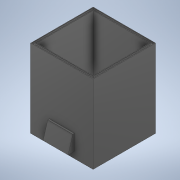
# Autodesk Inventor part: Bauteil1
Saved by Autodesk Inventor 2020 (Build 240168000, 168)
## iProperties
Created: 2021-04-07
Part Number: Bauteil1
Material: Acetalharz, Schwarz
Document SubType Name: Modeling
Designer: Julian Uhl
Density: 1.425 g/cm^3
Appearance: Glatt - Schwarz
Author: Julian Uhl
Autodesk Inventor part; units mm, degrees
ref_plane "YZ Plane" through (0, 0, 0) normal (1, 0, 0) x (0, 1, 0)
ref_plane "XZ Plane" through (0, 0, 0) normal (0, 1, 0) x (-1, 0, 0)
ref_plane "XY Plane" through (0, 0, 0) normal (0, 0, 1) x (1, 0, 0)
sketch "Skizze1" plane through (0, 0, 0) normal (0, 0, 1) x (1, 0, 0)
  line L0 (-140, 0) -> (140, 0) projected
  line L1 (0, -140) -> (0, 140) projected
  line L2 (-100, 100) -> (100, 100)
  line L3 (100, 100) -> (100, -100)
  line L4 (100, -100) -> (-100, -100)
  line L5 (-100, -100) -> (-100, 100)
  point P0 (0, 0)
  dimension "d0" = 200
  dimension "d1" = 200
  dimension "d2" = 100
  dimension "d3" = 100
  constraints: 8 end point, 2 parallel, 1 horizontal, 1 perpendicular
  measures "d0" distance between parallel lines of L3 L5
  measures "d1" distance between parallel lines of L4 L2
  measures "d2" distance between parallel lines of L0 L2
  measures "d3" distance between parallel lines of L1 L5
extrude "Extrusion1" add sketch "Skizze1" along normal blind 200
sketch "Skizze2" plane through (-100, 100, 0) normal (0, 1, 0) x (1, 0, 0)
  line L0 (10, -10) -> (190, -10)
  line L1 (190, -10) -> (190, -190)
  line L2 (190, -190) -> (10, -190)
  line L3 (10, -190) -> (10, -10)
  line L4 (0, 0) -> (0, -200) projected
  line L5 (200, 0) -> (200, -200) projected
  line L6 (200, -200) -> (0, -200) projected
  line L7 (200, 0) -> (0, 0) projected
  point P0 (100, 0)
  dimension "d6" = 10
  dimension "d7" = 10
  dimension "d8" = 10
  dimension "d9" = 10
  constraints: 8 end point, 2 parallel, 1 horizontal, 1 perpendicular
  measures "d6" distance between parallel lines of L3 L4
  measures "d7" distance between parallel lines of L5 L1
  measures "d8" distance between parallel lines of L6 L2
  measures "d9" distance between parallel lines of L0 L7
extrude "Extrusion2" cut sketch "Skizze2" against normal blind 190 contours L0 L1 L2 L3
sketch "Skizze3" plane through (-100, 100, 0) normal (0, 1, 0) x (1, 0, 0)
  line L0 (2, -2) -> (198, -2)
  line L1 (198, -2) -> (198, -198)
  line L2 (198, -198) -> (2, -198)
  line L3 (2, -198) -> (2, -2)
  line L4 (8, -8) -> (192, -8)
  line L5 (192, -8) -> (192, -192)
  line L6 (192, -192) -> (8, -192)
  line L7 (8, -192) -> (8, -8)
  line L8 (0, 0) -> (0, -200) projected
  line L9 (10, -190) -> (10, -10) projected
  line L10 (190, -190) -> (10, -190) projected
  line L11 (200, -200) -> (0, -200) projected
  line L12 (190, -10) -> (190, -190) projected
  line L13 (200, 0) -> (200, -200) projected
  line L14 (200, 0) -> (0, 0) projected
  line L15 (10, -10) -> (190, -10) projected
  point P0 (100, 0)
  dimension "d12" = 2
  dimension "d13" = 2
  dimension "d14" = 2
  dimension "d15" = 2
  dimension "d16" = 2
  dimension "d17" = 2
  dimension "d18" = 2
  dimension "d19" = 2
  constraints: 16 end point, 4 parallel, 2 horizontal, 2 perpendicular
  measures "d12" distance between parallel lines of L8 L3
  measures "d13" distance between parallel lines of L9 L7
  measures "d14" distance between parallel lines of L10 L6
  measures "d15" distance between parallel lines of L11 L2
  measures "d16" distance between parallel lines of L12 L5
  measures "d17" distance between parallel lines of L13 L1
  measures "d18" distance between parallel lines of L14 L0
  measures "d19" distance between parallel lines of L15 L4
extrude "Extrusion3" cut sketch "Skizze3" against normal blind 5 contours L0 L1 L2 L3
fillet "Rundung1" radius 0.5 8 edges at (0, 100, 2) (0, 100, 8) (98, 100, 100) (92, 100, 100) (0, 100, 192) (0, 100, 198) (-98, 100, 100) (-92, 100, 100)
sketch "Skizze5" plane through (-100, -90, 0) normal (0, 1, 0) x (1, 0, 0)
  line L0 (95, -95) -> (105, -95)
  line L1 (105, -95) -> (105, -105)
  line L2 (105, -105) -> (95, -105)
  line L3 (95, -105) -> (95, -95)
  line L4 (200, 0) -> (0, 0) projected
  line L5 (0, 0) -> (0, -200) projected
  point P0 (100, 0)
  dimension "d24" = 10
  dimension "d25" = 10
  dimension "d26" = 95
  dimension "d27" = 95
  constraints: 8 end point, 2 parallel, 1 horizontal, 1 perpendicular
  measures "d24" distance between parallel lines of L2 L0
  measures "d25" distance between parallel lines of L1 L3
  measures "d26" distance between parallel lines of L4 L0
  measures "d27" distance between parallel lines of L5 L3
extrude "Extrusion4" cut sketch "Skizze5" against normal blind 7
sketch "Skizze6" plane through (-100, -100, 0) normal (0, -1, 0) x (1, 0, 0)
  line L0 (10, 190) -> (190, 190)
  line L1 (190, 190) -> (190, 10)
  line L2 (190, 10) -> (10, 10)
  line L3 (10, 10) -> (10, 190)
  line L4 (0, 200) -> (200, 200) projected
  line L5 (200, 0) -> (200, 200) projected
  line L6 (0, 0) -> (200, 0) projected
  line L7 (0, 0) -> (0, 200) projected
  point P0 (100, 0)
  dimension "d30" = 10
  dimension "d31" = 10
  dimension "d32" = 10
  dimension "d33" = 10
  constraints: 8 end point, 2 parallel, 1 horizontal, 1 perpendicular
  measures "d30" distance between parallel lines of L4 L0
  measures "d31" distance between parallel lines of L5 L1
  measures "d32" distance between parallel lines of L6 L2
  measures "d33" distance between parallel lines of L7 L3
extrude "Extrusion5" add sketch "Skizze6" along normal blind 50
sketch "Skizze7" plane through (0, 0, 200) normal (0, 0, 1) x (1, 0, 0)
  line L0 (-40, -130) -> (40, -130)
  line L1 (40, -130) -> (40, -80)
  line L2 (40, -80) -> (-40, -80)
  line L3 (-40, -80) -> (-40, -130)
  line L4 (100, -150) -> (-100, -150) projected
  line L5 (-100, 100) -> (-100, -150) projected
  point P0 (0, 0)
  dimension "d36" = 50
  dimension "d37" = 80
  dimension "d38" = 20
  dimension "d39" = 60
  constraints: 8 end point, 2 parallel, 1 horizontal, 1 perpendicular
  measures "d36" distance of L2.end L0.start
  measures "d37" distance between parallel lines of L1 L3
  measures "d38" distance between parallel lines of L4 L0
  measures "d39" distance between parallel lines of L5 L3
extrude "Extrusion6" add sketch "Skizze7" along normal blind 20
sketch "Skizze9" plane through (-40, -130, 200) normal (-1, 0, 0) x (0, 0, 1)
  line L0 (20, 0) -> (20, 50) projected
  line L1 (20, 0) -> (5, 50)
  line L2 (0, 50) -> (20, 50) projected
  line L3 (0, 230) -> (0, -20) projected
  point P0 (-200, 130)
  dimension "d45" = 5
  constraints: 2 end point, 1 point on line
  measures "d45" distance from line of L1.end L3
extrude "Extrusion7" cut sketch "Skizze9" against normal blind 200
fillet "Rundung2" radius 2 4 edges at (0, -90, 10) (90, -90, 100) (0, -90, 190) (-90, -90, 100)
chamfer "Fase1" distance 1 angle 45 4 edges at (0, -90, 95) (5, -90, 100) (0, -90, 105) (-5, -90, 100)
